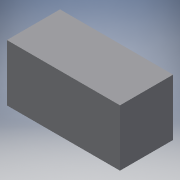
# Autodesk Inventor part: Side pontoon2
Saved by Autodesk Inventor 2018 (Build 220112000, 112)
## iProperties
Created: 2018-02-19
Part Number: Side pontoon2
Material: 一般
Document SubType Name: Modeling
Designer: kit
Density: 1 g/cm^3
Appearance: 既定
Author: kit
Autodesk Inventor part; units mm, degrees
ref_plane "YZ Plane" through (0, 0, 0) normal (1, 0, 0) x (0, 1, 0)
ref_plane "XZ Plane" through (0, 0, 0) normal (0, 1, 0) x (-1, 0, 0)
ref_plane "XY Plane" through (0, 0, 0) normal (0, 0, 1) x (1, 0, 0)
sketch "スケッチ1" plane through (0, 0, 0) normal (1, 0, 0) x (0, 1, 0)
  line L0 (-227, -51.5) -> (-697, -51.5)
  line L1 (-697, -51.5) -> (-697, -551.5)
  line L2 (-697, -551.5) -> (-227, -551.5)
  line L3 (-227, -551.5) -> (-227, -51.5)
  line L4 (-836.4, 0) -> (139.4, 0) projected
  line L5 (0, 110.3) -> (0, -661.8) projected
  point P0 (0, 0)
  dimension "d2" = 500
  dimension "d3" = 470
  dimension "d4" = 51.5
  dimension "d6" = 697
  constraints: 8 end point, 2 parallel, 1 horizontal, 1 perpendicular
  measures "d2" distance of L2.end L0.start
  measures "d3" distance of L0.start L0.end
  measures "d4" distance between parallel lines of L0 L4
  measures "d6" distance between parallel lines of L5 L1
extrude "押し出し1" add sketch "スケッチ1" along normal blind 1000
